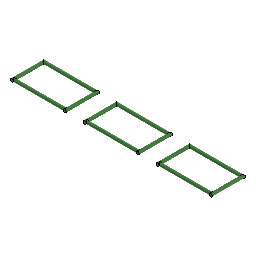
IRC_table (Autodesk Fusion 360 archive; units mm, degrees)
design "irc_goal"
Autodesk Fusion 360 part; units mm, degrees
sketch "スケッチ1" plane through (0, 0, 0) normal (0, 0, 1) x (1, 0, 0)
  line L0 (-49.9185, 0) -> (-49.9185, 300) construction
  line L1 (-49.9185, 300) -> (450.0815, 300) construction
  line L2 (450.0815, 300) -> (450.0815, 0) construction
  line L3 (-49.9185, 0) -> (450.0815, 0) construction
  line L4 (-35.9185, 0) -> (-35.9185, 286)
  line L5 (-35.9185, 286) -> (436.0815, 286)
  line L6 (436.0815, 286) -> (436.0815, 0)
  line L7 (-35.9185, 14) -> (436.0815, 14)
  line L8 (600.0815, 0) -> (600.0815, 300) construction
  line L9 (600.0815, 300) -> (1100.0815, 300) construction
  line L10 (1100.0815, 300) -> (1100.0815, 0) construction
  line L11 (1250.0815, 0) -> (1250.0815, 300) construction
  line L12 (1250.0815, 300) -> (1750.0815, 300) construction
  line L13 (1750.0815, 300) -> (1750.0815, 0) construction
  line L14 (614.0815, 0) -> (614.0815, 286)
  line L15 (614.0815, 286) -> (1086.0815, 286)
  line L16 (1086.0815, 286) -> (1086.0815, 0)
  line L17 (1264.0815, 0) -> (1264.0815, 286)
  line L18 (1264.0815, 286) -> (1736.0815, 286)
  line L19 (1736.0815, 286) -> (1736.0815, 0)
  line L20 (614.0815, 14) -> (1086.0815, 14)
  line L21 (1264.0815, 14) -> (1279.8524, 14)
  line L22 (1279.8524, 14) -> (1736.0815, 14)
  dimension "d1" = 300
  dimension "d2" = 500
  dimension "d15" = 500
  dimension "d16" = 500
  dimension "d17" = 650
  dimension "d18" = 650
  dimension "d19" = 14
  dimension "d20" = 14
  constraint vertical L0
  constraint perpendicular L0 L1
  constraint perpendicular L1 L2
  constraint coincident L4 L7.start
  constraint coincident L6 L7.end
  constraint perpendicular L1 L8
  constraint perpendicular L8 L9
  constraint perpendicular L9 L10
  constraint perpendicular L9 L11
  constraint perpendicular L10 L12
  constraint perpendicular L12 L13
  constraint coincident L14 L20.start
  constraint coincident L16 L20.end
  constraint perpendicular L16 L20
  constraint coincident L17 L21.start
  constraint perpendicular L17 L21
  constraint coincident L19 L22.end
  constraint perpendicular L13 L22
  measures "d1" distance of L0.start L0.end
  measures "d2" distance of L0.end L1.end
  measures "d15" distance of L8.end L9.end
  measures "d16" distance of L11.end L12.end
  measures "d17" distance of L0 L8
  measures "d18" distance of L8 L11
pipe "パイプ1" add diameter 28 path "スケッチ1" along L4 L5 L6 makes body 1
pipe "パイプ2" add diameter 28 path "スケッチ1" along L7 bodies 1
pipe "パイプ3" add diameter 28 path "スケッチ1" along L14 L15 L16 separate body makes body 2
pipe "パイプ4" add diameter 28 path "スケッチ1" along L17 L18 L19 separate body makes body 3
pipe "パイプ5" add diameter 28 path "スケッチ1" along L20 bodies 2
pipe "パイプ6" add diameter 28 path "スケッチ1" along L22 L21 bodies 3
